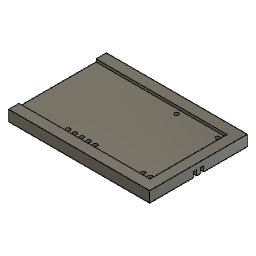
PCB v6 (Autodesk Fusion 360 design; units mm, degrees)
Autodesk Fusion 360 part; units mm, degrees
sketch "Skizze1" plane through (0, 0, 0) normal (0, 1, 0) x (1, 0, 0)
  line L0 (-26.25, 18.2) -> (26.25, 18.2)
  line L1 (26.25, 18.2) -> (26.25, -18.2)
  line L2 (26.25, -18.2) -> (-26.25, -18.2)
  line L3 (-26.25, -18.2) -> (-26.25, 18.2)
  line L4 (-26.25, 18.2) -> (26.25, -18.2) construction
  line L5 (-26.25, -18.2) -> (26.25, 18.2) construction
  dimension "d1" = 52.5
  dimension "d2" = 36.4
  constraint horizontal L0
  constraint vertical L1
  constraint horizontal L2
  constraint vertical L3
  constraint coincident origin L5
  constraint coincident origin L4
  measures "d1" distance of L0.start L0.end
  measures "d2" distance of L0.start L2.end
extrude "Extrude1" add sketch "Skizze1" along normal blind 4
sketch "ESP Pocket" plane through (0, 4, 0) normal (0, 1, 0) x (-1, 0, 0)
  line L0 (26.25, 18.2) -> (-26.25, 18.2)
  line L1 (-26.25, 18.2) -> (-26.25, -18.2)
  line L2 (-26.25, -18.2) -> (26.25, -18.2)
  line L3 (26.25, -18.2) -> (26.25, 18.2)
  line L4 (26.25, -14.35) -> (-22.55, -14.35)
  line L5 (-22.55, -14.35) -> (-22.55, 14.35)
  line L6 (-22.55, 14.35) -> (26.25, 14.35)
  line L7 (26.25, 14.35) -> (26.25, -14.35)
  line L8 (-22.55, -14.35) -> (-26.25, -18.2) construction
  line L9 (-22.55, 14.35) -> (-26.25, 18.2) construction
  dimension "d12" = 48.8
  dimension "d13" = 28.7
  constraint horizontal L4
  constraint vertical L5
  constraint horizontal L6
  constraint vertical L7
  constraint coincident L3 L4.start
  constraint coincident L1.end L2.start
  constraint coincident L0.end L1.start
  constraint equal L8 L9
  measures "d12" distance of L4.start L4.end
  measures "d13" distance of L4.end L5.end
extrude "Extrude2" cut sketch "ESP Pocket" against normal blind 1 contours L3 L4 L5 L6 L7
sketch "Pin Holes" plane through (0, 3, 0) normal (0, 1, 0) x (-1, 0, 0)
  line L0 (26.25, 14.35) -> (-22.55, 14.35)
  line L1 (-22.55, 14.35) -> (-22.55, -14.35)
  line L2 (-22.55, -14.35) -> (26.25, -14.35)
  line L3 (26.25, -14.35) -> (26.25, 14.35)
  circle A0 centre (-20.8, -12.6) radius 0.75
  circle A1 centre (-20.8, 12.6) radius 0.75
  circle A2 centre (-18.26, 12.6) radius 0.75
  circle A3 centre (-0.48, 12.6) radius 0.75
  circle A4 centre (2.06, 12.6) radius 0.75
  circle A5 centre (4.6, 12.6) radius 0.75
  circle A6 centre (7.14, 12.6) radius 0.75
  circle A7 centre (9.68, 12.6) radius 0.75
  circle A8 centre (-5.56, -12.6) radius 0.75
  dimension "d20" = 1.5
  dimension "d21" = 1.75
  dimension "d22" = 1.75
  dimension "d27" = 1.5
  dimension "d28" = 1.75
  dimension "d29" = 1.75
  dimension "d32" = 2.54
  dimension "d33" = 0
  dimension "d40" = 2.54
  dimension "d41" = 0
  measures "d20" diameter of A0
  measures "d21" distance of L1 A0.centre
  measures "d22" distance of L2 A0.centre
  measures "d27" diameter of A1
  measures "d28" distance of L1 A1.centre
  measures "d29" distance of L0 A1.centre
extrude "Extrude3" cut sketch "Pin Holes" against normal up to surface (3 mm away) contours A0 | A1 | A2 | A3 | A4 | A5 | A6 | A7 | A8
sketch "Power Pin Holes" plane through (26.25, 0, 0) normal (1, 0, 0) x (0, 0, -1)
  line L0 (-18.2, 0) -> (18.2, 0)
  line L1 (18.2, 0) -> (18.2, 4)
  line L2 (18.2, 4) -> (-18.2, 4)
  line L3 (-18.2, 4) -> (-18.2, 0)
  line L4 (-1.92, 2) -> (-0.62, 2)
  line L5 (-0.62, 2) -> (-0.62, 0)
  line L6 (-0.62, 0) -> (-1.92, 0)
  line L7 (-1.92, 0) -> (-1.92, 2)
  line L8 (0.62, 0) -> (1.92, 0)
  line L9 (1.92, 0) -> (1.92, 2)
  line L10 (1.92, 2) -> (0.62, 2)
  line L11 (0.62, 2) -> (0.62, 0)
  line L12 (-0.62, 2) -> (0, 0) construction
  line L13 (0.62, 2) -> (0, 0) construction
  dimension "d44" = 2
  dimension "d45" = 2
  dimension "d46" = 1.3
  dimension "d47" = 1.3
  dimension "d48" = 2.54
  constraint horizontal L4
  constraint vertical L5
  constraint horizontal L6
  constraint vertical L7
  constraint coincident L0 L5.end
  constraint horizontal L8
  constraint vertical L9
  constraint horizontal L10
  constraint vertical L11
  constraint coincident L0 L8.start
  constraint coincident L12.end L13.end
  constraint equal L12 L13
  measures "d44" distance of L4.start L6.end
  measures "d45" distance of L8.end L9.end
  measures "d46" distance of L4.start L4.end
  measures "d47" distance of L9.end L10.end
  measures "d48" distance of L6.end L8.start
extrude "Extrude4" cut sketch "Power Pin Holes" against normal blind 6 contours L0 L4 L5 L6 L7 | L0 L8 L9 L10 L11
sketch "Data Pin Holes" plane through (0, 0, -18.2) normal (0, 0, -1) x (-1, 0, 0)
  line L0 (-26.25, 0) -> (26.25, 0)
  line L1 (26.25, 0) -> (26.25, 4)
  line L2 (26.25, 4) -> (-26.25, 4)
  line L3 (-26.25, 4) -> (-26.25, 0)
  line L4 (-6.21, 2) -> (-4.91, 2)
  line L5 (-4.91, 2) -> (-4.91, 0)
  line L6 (-4.91, 0) -> (-6.21, 0)
  line L7 (-6.21, 0) -> (-6.21, 2)
  line L8 (-6.31, 3) -> (-4.81, 3)
  line L9 (-6.21, 2) -> (-6.31, 3) construction
  line L10 (-4.81, 3) -> (-4.91, 2) construction
  line L11 (22.25, 0) -> (20.95, 0)
  line L12 (20.95, 0) -> (20.95, 2)
  line L13 (20.95, 2) -> (22.25, 2)
  line L14 (22.25, 2) -> (22.25, 0)
  line L15 (18.41, 0) -> (18.41, 2)
  line L16 (18.41, 2) -> (19.71, 2)
  line L17 (19.71, 2) -> (19.71, 0)
  line L18 (19.71, 0) -> (18.41, 0)
  line L19 (15.87, 0) -> (15.87, 2)
  line L20 (15.87, 2) -> (17.17, 2)
  line L21 (17.17, 2) -> (17.17, 0)
  line L22 (17.17, 0) -> (15.87, 0)
  line L23 (13.33, 0) -> (13.33, 2)
  line L24 (13.33, 2) -> (14.63, 2)
  line L25 (14.63, 2) -> (14.63, 0)
  line L26 (14.63, 0) -> (13.33, 0)
  line L27 (10.79, 0) -> (10.79, 2)
  line L28 (10.79, 2) -> (12.09, 2)
  line L29 (12.09, 2) -> (12.09, 0)
  line L30 (12.09, 0) -> (10.79, 0)
  line L31 (8.25, 0) -> (8.25, 2)
  line L32 (8.25, 2) -> (9.55, 2)
  line L33 (9.55, 2) -> (9.55, 0)
  line L34 (9.55, 0) -> (8.25, 0)
  line L35 (5.71, 0) -> (5.71, 2)
  line L36 (5.71, 2) -> (7.01, 2)
  line L37 (7.01, 2) -> (7.01, 0)
  line L38 (7.01, 0) -> (5.71, 0)
  line L39 (3.17, 0) -> (3.17, 2)
  line L40 (3.17, 2) -> (4.47, 2)
  line L41 (4.47, 2) -> (4.47, 0)
  line L42 (4.47, 0) -> (3.17, 0)
  dimension "d51" = 1.3
  dimension "d52" = 2
  dimension "d55" = 1.3
  dimension "d56" = 2
  dimension "d57" = 4
  dimension "d60" = -2.54
  dimension "d61" = 0
  constraint horizontal L4
  constraint vertical L5
  constraint horizontal L6
  constraint vertical L7
  constraint coincident L0 L5.end
  constraint coincident L8.start L9.end
  constraint coincident L8.end L10.start
  constraint equal L9 L10
  constraint horizontal L11
  constraint vertical L12
  constraint horizontal L13
  constraint vertical L14
  constraint coincident L0 L11.start
  measures "d51" distance of L4.start L4.end
  measures "d52" distance of L4.start L6.end
  measures "d55" distance of L12.end L13.end
  measures "d56" distance of L11.end L12.end
  measures "d57" distance of L1 L11.start
extrude "Extrude5" cut sketch "Data Pin Holes" against normal blind 6 contours L0 L4 L5 L6 L7
extrude "Extrude6" cut sketch "Data Pin Holes" against normal blind 6 contours L0 L39 L40 L41 L42 | L0 L11 L12 L13 L14 | L0 L35 L36 L37 L38 | L0 L15 L16 L17 L18 | L0 L31 L32 L33 L34 | L0 L19 L20 L21 L22 | L0 L27 L28 L29 L30 | L0 L23 L24 L25 L26
sketch "Circuit Lanes" plane through (0, 0, 0) normal (0, -1, 0) x (1, 0, 0)
  circle A0 centre (-9.68, 12.6) radius 0.75
  circle A1 centre (0.48, 12.6) radius 0.75
  circle A2 centre (18.26, 12.6) radius 0.75
  circle A3 centre (-7.14, 12.6) radius 0.75
  circle A4 centre (-2.06, 12.6) radius 0.75
  circle A5 centre (20.8, -12.6) radius 0.75
  circle A6 centre (20.8, 12.6) radius 0.75
  circle A7 centre (-4.6, 12.6) radius 0.75
  line L0 (-17.17, -18.2) -> (-17.17, -12.2)
  line L1 (-9.55, -12.2) -> (-8.25, -12.2)
  line L2 (-15.87, -12.2) -> (-15.87, -18.2)
  line L3 (-8.25, -18.2) -> (-7.01, -18.2)
  line L4 (-14.63, -18.2) -> (-14.63, -12.2)
  line L5 (-14.63, -12.2) -> (-13.33, -12.2)
  line L6 (-13.33, -12.2) -> (-13.33, -18.2)
  line L7 (-13.33, -18.2) -> (-12.09, -18.2)
  line L8 (4.91, -18.2) -> (4.91, -12.9742)
  arc A8 (4.91, -12.2258) -> (4.91, -12.9742) centre (5.56, -12.6) ccw
  line L9 (6.21, -12.2) -> (6.21, -12.2258)
  line L10 (6.21, -18.2) -> (26.25, -18.2)
  line L11 (26.25, -18.2) -> (26.25, -1.92)
  line L12 (26.25, -1.92) -> (20.25, -1.92)
  line L13 (20.25, -1.92) -> (20.25, -0.62)
  line L14 (20.25, -0.62) -> (26.25, -0.62)
  line L15 (26.25, -0.62) -> (26.25, 0.62)
  line L16 (26.25, 0.62) -> (20.25, 0.62)
  line L17 (20.25, 0.62) -> (20.25, 1.92)
  line L18 (20.25, 1.92) -> (26.25, 1.92)
  line L19 (26.25, 1.92) -> (26.25, 18.2)
  line L20 (26.25, 18.2) -> (-26.25, 18.2)
  line L21 (-26.25, 18.2) -> (-26.25, -18.2)
  line L22 (-26.25, -18.2) -> (-22.25, -18.2)
  line L23 (-22.25, -18.2) -> (-22.25, -12.2)
  line L24 (-22.25, -12.2) -> (-20.95, -12.2)
  line L25 (-20.95, -12.2) -> (-20.95, -18.2)
  line L26 (-20.95, -18.2) -> (-19.71, -18.2)
  line L27 (-19.71, -18.2) -> (-19.71, -12.2)
  line L28 (-19.71, -12.2) -> (-18.41, -12.2)
  line L29 (-18.41, -12.2) -> (-18.41, -18.2)
  line L30 (-18.41, -18.2) -> (-17.17, -18.2)
  line L31 (20.3, 12.6) -> (21.3, 12.6)
  line L32 (21.3, 12.6) -> (21.3, 1.92)
  line L33 (20.3, -12.6) -> (21.3, -12.6)
  line L34 (21.3, -12.6) -> (21.3, -1.92)
  line L35 (-9.55, -18.2) -> (-9.55, -12.2)
  line L36 (-8.25, -12.2) -> (-8.25, -18.2)
  line L37 (-7.01, -18.2) -> (-7.01, -12.2)
  line L38 (-7.01, -12.2) -> (-5.71, -12.2)
  line L39 (-5.71, -12.2) -> (-5.71, -18.2)
  line L40 (-5.71, -18.2) -> (-4.47, -18.2)
  line L41 (-4.47, -18.2) -> (-4.47, -12.2)
  line L42 (-4.47, -12.2) -> (-3.17, -12.2)
  line L43 (-3.17, -12.2) -> (-3.17, -18.2)
  line L44 (-3.17, -18.2) -> (4.91, -18.2)
  line L45 (-12.09, -18.2) -> (-12.09, -12.2)
  line L46 (-12.09, -12.2) -> (-10.79, -12.2)
  line L47 (-10.79, -12.2) -> (-10.79, -18.2)
  line L48 (-10.79, -18.2) -> (-9.55, -18.2)
  line L49 (-4.32, -12.2) -> (-4.32, -6.7498)
  line L50 (-4.32, -6.7498) -> (-2.1481, -4.5615)
  line L51 (-2.1481, -4.5615) -> (18.3548, -4.5615)
  line L52 (18.3548, -5.5615) -> (-1.7317, -5.5615)
  line L53 (-1.7317, -5.5615) -> (-3.32, -7.1618)
  line L54 (-3.32, -7.1618) -> (-3.32, -12.2)
  line L55 (-3.32, -12.2) -> (-4.32, -12.2)
  line L56 (-5.86, -12.2) -> (-5.86, -6.8818)
  line L57 (-5.86, -6.8818) -> (5.89, 4.9567)
  line L58 (5.89, 4.9567) -> (18.3548, 4.9567)
  line L59 (18.3548, 5.9567) -> (5.4736, 5.9567)
  line L60 (5.4736, 5.9567) -> (-6.86, -6.4698)
  line L61 (-6.86, -6.4698) -> (-6.86, -12.2)
  line L62 (-6.86, -12.2) -> (-5.86, -12.2)
  line L63 (-9.4, -12.2) -> (-8.4, -12.2)
  line L64 (-8.4, -12.2) -> (-8.4, -6.6018)
  line L65 (-8.4, -6.6018) -> (10.162, 12.1)
  line L66 (10.162, 12.1) -> (18.26, 12.1)
  line L67 (18.26, 12.1) -> (18.26, 13.1)
  line L68 (18.26, 13.1) -> (9.7456, 13.1)
  line L69 (9.7456, 13.1) -> (-9.4, -6.1898)
  line L70 (-9.4, -6.1898) -> (-9.4, -12.2)
  line L71 (-10.94, -12.2) -> (-10.94, -6.3219)
  line L72 (-10.94, -6.3219) -> (0.98, 5.6879)
  line L73 (0.98, 5.6879) -> (0.98, 12.6)
  line L74 (0.98, 12.6) -> (-0.02, 12.6)
  line L75 (-0.02, 12.6) -> (-0.02, 6.0999)
  line L76 (-0.02, 6.0999) -> (-11.94, -5.9099)
  line L77 (-11.94, -5.9099) -> (-11.94, -12.2)
  line L78 (-11.94, -12.2) -> (-10.94, -12.2)
  line L79 (-13.48, -12.2) -> (-13.48, -6.0419)
  line L80 (-13.48, -6.0419) -> (-1.56, 5.9679)
  line L81 (-1.56, 5.9679) -> (-1.56, 12.6)
  line L82 (-1.56, 12.6) -> (-2.56, 12.6)
  line L83 (-2.56, 12.6) -> (-2.56, 6.3799)
  line L84 (-2.56, 6.3799) -> (-14.48, -5.6299)
  line L85 (-14.48, -5.6299) -> (-14.48, -12.2)
  line L86 (-14.48, -12.2) -> (-13.48, -12.2)
  line L87 (-16.02, -12.2) -> (-16.02, -5.7619)
  line L88 (-16.02, -5.7619) -> (-4.1, 6.2478)
  line L89 (-4.1, 6.2478) -> (-4.1, 12.6)
  line L90 (-4.1, 12.6) -> (-5.1, 12.6)
  line L91 (-5.1, 12.6) -> (-5.1, 6.6599)
  line L92 (-5.1, 6.6599) -> (-17.02, -5.3499)
  line L93 (-17.02, -5.3499) -> (-17.02, -12.2)
  line L94 (-17.02, -12.2) -> (-16.02, -12.2)
  line L95 (-17.17, -12.2) -> (-15.87, -12.2)
  line L96 (-19.56, -12.2) -> (-18.56, -12.2)
  line L97 (-18.56, -12.2) -> (-18.56, -5.482)
  line L98 (-18.56, -5.482) -> (-6.64, 6.5278)
  line L99 (-6.64, 6.5278) -> (-6.64, 12.6)
  line L100 (-6.64, 12.6) -> (-7.64, 12.6)
  line L101 (-7.64, 12.6) -> (-7.64, 6.9398)
  line L102 (-7.64, 6.9398) -> (-19.56, -5.0699)
  line L103 (-19.56, -5.0699) -> (-19.56, -12.2)
  line L104 (-9.18, 6.8078) -> (-9.18, 12.6)
  line L105 (-9.18, 12.6) -> (-10.18, 12.6)
  line L106 (-10.18, 12.6) -> (-10.18, 7.2198)
  line L107 (-10.18, 7.2198) -> (-22.1, -4.79)
  line L108 (-22.1, -4.79) -> (-22.1, -12.2)
  line L109 (-22.1, -12.2) -> (-21.1, -12.2)
  line L110 (-21.1, -12.2) -> (-21.1, -5.202)
  line L111 (-21.1, -5.202) -> (-9.18, 6.8078)
  line L112 (20.3, -1.92) -> (20.3, -3.4384)
  line L113 (20.3, -6.6845) -> (20.3, -12.6)
  line L114 (20.3, 1.92) -> (20.3, 3.8337)
  line L115 (20.3, 7.0798) -> (20.3, 12.6)
  line L116 (4.91, -12.2258) -> (4.91, -12.2)
  line L117 (4.91, -12.2) -> (4.9256, -12.2)
  arc A9 (6.1944, -12.2) -> (4.9256, -12.2) centre (5.56, -12.6) ccw
  line L118 (6.1944, -12.2) -> (6.21, -12.2)
  arc A10 (6.21, -12.9742) -> (6.21, -12.2258) centre (5.56, -12.6) ccw
  line L119 (6.21, -12.9742) -> (6.21, -18.2)
  line L120 (-17.17, -12.2) -> (-15.87, -12.2)
  line L121 (-15.87, -18.2) -> (-14.63, -18.2)
  line L122 (18.3548, 5.9567) -> (20.3, 7.0798)
  line L123 (18.3548, 4.9567) -> (20.3, 3.8337)
  line L124 (18.3548, -4.5615) -> (20.3, -3.4384)
  line L125 (18.3548, -5.5615) -> (20.3, -6.6845)
  dimension "d64" = 1
  dimension "d67" = 1
  dimension "d68" = 1
  dimension "d70" = 1
  dimension "d72" = 1
  dimension "d73" = 1
  dimension "d74" = 1
  dimension "d75" = 1
  dimension "d76" = 1
  dimension "d77" = 1
  dimension "d78" = 1
  dimension "d79" = 1
  dimension "d80" = 1
  dimension "d81" = 1
  dimension "d82" = 1
  dimension "d83" = 1
  dimension "d84" = 1
  dimension "d85" = 1
  dimension "d86" = 1
  dimension "d87" = 1
  dimension "d88" = 1
  dimension "d89" = 1
  dimension "d90" = 1
  dimension "d91" = 1
  dimension "d92" = 1
  dimension "d93" = 1
  dimension "d94" = 1
  dimension "d95" = 1
  dimension "d96" = 1
  dimension "d97" = 1
  dimension "d98" = 1
  dimension "d99" = 1
  dimension "d105" = 1
  constraint horizontal L31
  constraint vertical L32
  constraint vertical L114
  constraint coincident L18 L32.end
  constraint midpoint A6.centre L31
  constraint vertical L112
  constraint horizontal L33
  constraint vertical L34
  constraint coincident L12 L34.end
  constraint midpoint A5.centre L33
  constraint perpendicular L42 L49
  constraint perpendicular L51 L112
  constraint perpendicular L52 L112
  constraint parallel L50 L53
  constraint perpendicular L52 L54
  constraint horizontal L55
  constraint midpoint L42 L55
  constraint vertical L56
  constraint perpendicular L56 L58
  constraint perpendicular L56 L59
  constraint parallel L57 L60
  constraint perpendicular L58 L61
  constraint perpendicular L56 L62
  constraint parallel L50 L57
  constraint midpoint L38 L62
  constraint horizontal L63
  constraint perpendicular L63 L64
  constraint perpendicular L64 L66
  constraint perpendicular L66 L67
  constraint perpendicular L67 L68
  constraint vertical L70
  constraint parallel L60 L65
  constraint midpoint A2.centre L67
  constraint midpoint L1 L63
  constraint vertical L71
  constraint parallel L71 L73
  constraint perpendicular L71 L74
  constraint perpendicular L74 L75
  constraint parallel L72 L76
  constraint parallel L75 L77
  constraint horizontal L78
  constraint parallel L69 L72
  constraint parallel L65 L69
  constraint midpoint L46 L78
  constraint midpoint A1.centre L74
  constraint vertical L79
  constraint parallel L79 L81
  constraint perpendicular L79 L82
  constraint perpendicular L82 L83
  constraint parallel L80 L84
  constraint parallel L83 L85
  constraint horizontal L86
  constraint midpoint L5 L86
  constraint midpoint A4.centre L82
  constraint vertical L87
  constraint parallel L87 L89
  constraint perpendicular L87 L90
  constraint perpendicular L90 L91
  constraint parallel L88 L92
  constraint parallel L91 L93
  constraint horizontal L94
  constraint parallel L84 L88
  constraint midpoint L94 L95
  constraint midpoint A7.centre L90
  constraint vertical L97
  constraint parallel L97 L99
  constraint perpendicular L97 L100
  constraint perpendicular L100 L101
  constraint parallel L98 L102
  constraint parallel L101 L103
  constraint horizontal L96
  constraint vertical L110
  constraint parallel L104 L110
  constraint perpendicular L105 L110
  constraint perpendicular L105 L106
  constraint parallel L107 L111
  constraint parallel L106 L108
  constraint horizontal L109
  constraint parallel L92 L98
  constraint parallel L102 L111
  constraint midpoint L28 L96
  constraint midpoint A3.centre L100
  constraint midpoint A0.centre L105
  constraint midpoint L24 L109
  constraint collinear L112 L113
  constraint collinear L114 L115
  measures "d64" distance of L31.start L31.end
  measures "d67" distance of L33.start L33.end
  measures "d68" distance of L49.start L54.end
  measures "d70" distance of L50 L52.end
  measures "d72" distance of L57 L59.end
  measures "d73" distance of L56.start L61.end
  measures "d74" distance of L50 L57
  measures "d75" distance of L63.start L63.end
  measures "d76" distance of L64.end L69
  measures "d77" distance of L66.end L67.end
  measures "d78" distance of L60 L65
  measures "d79" distance of L73.end L74.end
  measures "d80" distance of L72 L75.end
  measures "d81" distance of L71.start L77.end
  measures "d82" distance of L69 L72
  measures "d83" distance of L81.end L82.end
  measures "d84" distance of L83.end L80
  measures "d85" distance of L79.start L85.end
  measures "d86" distance of L76 L80
  measures "d87" distance of L90.end L89.end
  measures "d88" distance of L91.end L88
  measures "d89" distance of L93.end L87.start
  measures "d90" distance of L84 L88
  measures "d91" distance of L100.end L99.end
  measures "d92" distance of L101.end L98
  measures "d93" distance of L96.end L96.start
  measures "d94" distance of L105.end L104.end
  measures "d95" distance of L106.end L111
  measures "d96" distance of L108.end L109.end
  measures "d97" distance of L92 L98
  measures "d98" distance of L102 L111
  measures "d99" distance of L58 L59
  measures "d105" distance of L51 L52
extrude "Extrude7" cut sketch "Circuit Lanes" against normal blind 1 contours A0 L24 L104 L106 L107 L108 L109 L110 L111 | A3 L28 L96 L97 L98 L99 L101 L102 L103 | A6 L18 L32 L38 L56 L57 L58 L59 L60 L61 L62 L114 L115 L122 L123 | A7 L87 L88 L89 L91 L92 L93 L94 L95 L120 | A5 L12 L34 L42 L49 L50 L51 L52 L53 L54 L55 L112 L113 L124 L125 | A4 L5 L79 L80 L81 L83 L84 L85 L86 | A2 L1 L63 L64 L65 L66 L68 L69 L70 | A1 L46 L71 L72 L73 L75 L76 L77 L78
equation "d1 = PCB_ESP_LENGTH + PCB_PADDING"
equation "d2 = PCB_ESP_WIDTH + PCB_PADDING * 2"
equation "PCB_ESP_LENGTH = 48.5 mm" comment "Length of the ESP dev board"
equation "PCB_ESP_WIDTH = 28.4 mm"
equation "PCB_DEPTH = 4 mm"
equation "PCB_PADDING = 4 mm"
equation "PCB_SOCKET_PIN_HOLE = 1.3 mm"
equation "PCB_3D_PRINT_TOLERANCE = 0.3 mm"
equation "PCB_CIRCUIT_LANE = 1 mm"
equation "d10 = PCB_DEPTH"
equation "d12 = PCB_ESP_LENGTH + PCB_3D_PRINT_TOLERANCE"
equation "d13 = PCB_ESP_WIDTH + PCB_3D_PRINT_TOLERANCE"
equation "d46 = PCB_SOCKET_PIN_HOLE"
equation "d47 = PCB_SOCKET_PIN_HOLE"
equation "d51 = PCB_SOCKET_PIN_HOLE"
equation "d55 = PCB_SOCKET_PIN_HOLE"
equation "d64 = PCB_CIRCUIT_LANE"
equation "d67 = PCB_CIRCUIT_LANE"
equation "d68 = PCB_CIRCUIT_LANE"
equation "d70 = PCB_CIRCUIT_LANE"
equation "d72 = PCB_CIRCUIT_LANE"
equation "d73 = PCB_CIRCUIT_LANE"
equation "d75 = PCB_CIRCUIT_LANE"
equation "d76 = PCB_CIRCUIT_LANE"
equation "d77 = PCB_CIRCUIT_LANE"
equation "d79 = PCB_CIRCUIT_LANE"
equation "d80 = PCB_CIRCUIT_LANE"
equation "d81 = PCB_CIRCUIT_LANE"
equation "d83 = PCB_CIRCUIT_LANE"
equation "d84 = PCB_CIRCUIT_LANE"
equation "d85 = PCB_CIRCUIT_LANE"
equation "d87 = PCB_CIRCUIT_LANE"
equation "d88 = PCB_CIRCUIT_LANE"
equation "d89 = PCB_CIRCUIT_LANE"
equation "d91 = PCB_CIRCUIT_LANE"
equation "d92 = PCB_CIRCUIT_LANE"
equation "d93 = PCB_CIRCUIT_LANE"
equation "d94 = PCB_CIRCUIT_LANE"
equation "d95 = PCB_CIRCUIT_LANE"
equation "d96 = PCB_CIRCUIT_LANE"
equation "d99 = PCB_CIRCUIT_LANE"
equation "d105 = PCB_CIRCUIT_LANE"
named bodies: "Body_PCB_ESP32"
